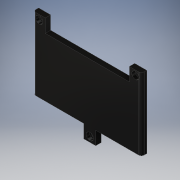
# Autodesk Inventor part: battery_cover
Saved by Autodesk Inventor 2019.4 (Build 234330000, 330)
## iProperties
Created: 2020-07-20
Part Number: battery_cover
Material: Generic
Document SubType Name: Modeling
Designer: alex_
Density: 1 g/cm^3
Appearance: Smooth - Black
Author: alex_
## iProperties of the stored document _3DPrint.ipt
Created: 2020-07-20
Part Number: _3DPrint
Material: Generic
Document SubType Name: Modeling
Designer: alex_
Density: 1 g/cm^3
Appearance: Default
Author: alex_
Autodesk Inventor part; units mm, degrees
ref_plane "YZ Plane" through (0, 0, 0) normal (1, 0, 0) x (0, 1, 0)
ref_plane "XZ Plane" through (0, 0, 0) normal (0, 1, 0) x (-1, 0, 0)
ref_plane "XY Plane" through (0, 0, 0) normal (0, 0, 1) x (1, 0, 0)
sketch "Sketch1" plane through (0, 0, 0) normal (0, 0, 1) x (1, 0, 0)
  line L0 (82, 0) -> (82, 45)
  line L1 (0, 45) -> (0, 0)
  line L2 (10, 45) -> (10, 55)
  line L3 (10, 55) -> (0, 55)
  line L4 (0, 55) -> (0, 45)
  line L5 (72, 45) -> (72, 55)
  line L6 (72, 55) -> (82, 55)
  line L7 (82, 55) -> (82, 45)
  line L8 (10, 45) -> (72, 45)
  line L9 (0, 0) -> (37.791, 0)
  line L10 (37.791, 0) -> (37.791, -10)
  line L11 (37.791, -10) -> (47.791, -10)
  line L12 (47.791, -10) -> (47.791, 0)
  line L13 (47.791, 0) -> (82, 0)
  circle A0 centre (42.843, -5.687) radius 1.6
  line L14 (0, 45) -> (0, 51)
  line L15 (82, 45) -> (82, 51)
  circle A1 centre (4.971, 51) radius 1.6
  circle A2 centre (77.029, 51) radius 1.6
  dimension "d0" = 82
  dimension "d1" = 45
  dimension "d2" = 10
  dimension "d3" = 10
  dimension "d4" = 10
  dimension "d5" = 10
  dimension "d10" = 37.791
  dimension "d11" = 10
  dimension "d12" = 10
  dimension "d15" = 3.2
  dimension "d16" = 6
  dimension "d20" = 3.2
  dimension "d21" = 3.2
  constraints: 32 end point, 4 perpendicular, 3 centre point, 3 parallel, 3 point on line, 2 horizontal
  measures "d0" distance of L1.start L0.end
  measures "d1" distance of L0.end L0.start
  measures "d2" distance of L3.end L2.end
  measures "d3" distance of L2.end L2.start
  measures "d4" distance of L5.end L6.end
  measures "d5" distance of L5.start L5.end
  measures "d10" distance of L1.end L9.end
  measures "d11" distance of L9.end L10.end
  measures "d12" distance of L10.end L11.end
  measures "d15" diameter of A0
  measures "d16" distance of L1.start L14.end
  measures "d20" diameter of A1
  measures "d21" diameter of A2
extrude "Extrusion1" add sketch "Sketch1" along normal blind 4
sketch "Sketch3" plane through (0, 0, 4) normal (0, 0, 1) x (1, 0, 0)
  circle A0 centre (4.971, 51) radius 1.6 projected
  circle A1 centre (4.971, 51) radius 2.75
  circle A2 centre (77.029, 51) radius 1.6 projected
  circle A3 centre (77.029, 51) radius 2.75
  circle A4 centre (42.843, -5.687) radius 1.6 projected
  circle A5 centre (42.843, -5.687) radius 2.75
  point P0 (0, 0)
  dimension "d24" = 5.5
  dimension "d25" = 5.5
  dimension "d26" = 5.5
  constraints: 3 centre point, 3 coincident
  measures "d24" diameter of A1
  measures "d25" diameter of A3
  measures "d26" diameter of A5
extrude "Extrusion2" cut sketch "Sketch3" against normal blind 2.5
sketch "Sketch4" plane through (0, 0, 4) normal (0, 0, 1) x (1, 0, 0)
  line L0 (10, 55) -> (0, 55) projected
  line L1 (10, 45) -> (10, 55) projected
  line L2 (0, 55) -> (10, 55)
  line L3 (10, 55) -> (10, 54.5)
  line L4 (10, 54.5) -> (0, 54.5)
  line L5 (0, 54.5) -> (0, 55)
  line L6 (0, 0) -> (0, 55) projected
  line L7 (0, 0) -> (37.791, 0) projected
  line L8 (0, 55) -> (0.5, 55)
  line L9 (0.5, 55) -> (0.5, 0)
  line L10 (0.5, 0) -> (0, 0)
  line L11 (0, 0) -> (0, 55)
  line L12 (0, 0) -> (37.791, 0)
  line L13 (37.791, 0) -> (37.791, 0.5)
  line L14 (37.791, 0.5) -> (0, 0.5)
  line L15 (0, 0.5) -> (0, 0)
  line L16 (37.791, 0) -> (37.791, -10) projected
  line L17 (37.791, -10) -> (38.291, -10)
  line L18 (38.291, -10) -> (38.291, 0.5)
  line L19 (38.291, 0.5) -> (37.791, 0.5)
  line L20 (37.791, 0.5) -> (37.791, -10)
  line L21 (47.791, 0) -> (47.791, -10) projected
  line L22 (37.791, -10) -> (47.791, -10)
  line L23 (47.791, -10) -> (47.791, -9.5)
  line L24 (47.791, -9.5) -> (37.791, -9.5)
  line L25 (37.791, -9.5) -> (37.791, -10)
  line L26 (47.791, -10) -> (47.291, -10)
  line L27 (47.291, -10) -> (47.291, 0.5)
  line L28 (47.291, 0.5) -> (47.791, 0.5)
  line L29 (47.791, 0.5) -> (47.791, -10)
  line L30 (82, 0) -> (82, 55) projected
  line L31 (47.291, 0.5) -> (82, 0.5)
  line L32 (82, 0.5) -> (82, 0)
  line L33 (82, 0) -> (47.291, 0)
  line L34 (47.291, 0) -> (47.291, 0.5)
  line L35 (82, 55) -> (72, 55) projected
  line L36 (82, 0) -> (81.5, 0)
  line L37 (81.5, 0) -> (81.5, 55)
  line L38 (81.5, 55) -> (82, 55)
  line L39 (82, 55) -> (82, 0)
  line L40 (72, 55) -> (72, 45) projected
  line L41 (82, 55) -> (72, 55)
  line L42 (72, 55) -> (72, 54.5)
  line L43 (72, 54.5) -> (82, 54.5)
  line L44 (82, 54.5) -> (82, 55)
  line L45 (10, 45) -> (72, 45) projected
  line L46 (10, 45) -> (72, 45)
  line L47 (72, 45) -> (72, 44.5)
  line L48 (72, 44.5) -> (10, 44.5)
  line L49 (10, 44.5) -> (10, 45)
  line L50 (72, 44.5) -> (72.5, 44.5)
  line L51 (72.5, 44.5) -> (72.5, 55)
  line L52 (72.5, 55) -> (72, 55)
  line L53 (72, 55) -> (72, 44.5)
  line L54 (10, 44.5) -> (9.5, 44.5)
  line L55 (9.5, 44.5) -> (9.5, 55)
  line L56 (9.5, 55) -> (10, 55)
  line L57 (10, 55) -> (10, 44.5)
  dimension "d30" = 0.5
  dimension "d31" = 0.5
  dimension "d32" = 0.5
  dimension "d33" = 0.5
  dimension "d34" = 0.5
  dimension "d35" = 0.5
  dimension "d36" = 0.5
  dimension "d37" = 0.5
  dimension "d38" = 0.5
  dimension "d39" = 0.5
  dimension "d40" = 0.5
  constraints: 96 end point, 24 parallel, 12 horizontal, 12 perpendicular, 9 point on line
  measures "d30" distance of L2.end L3.end
  measures "d31" distance of L9.end L10.end
  measures "d32" distance of L13.end L12.end
  measures "d33" distance of L19.end L18.end
  measures "d34" distance of L23.end L22.end
  measures "d35" distance of L27.end L28.end
  measures "d36" distance of L37.end L38.end
  measures "d37" distance of L42.end L41.end
  measures "d38" distance of L46.end L47.end
  measures "d39" distance of L52.end L51.end
  measures "d40" distance of L55.end L56.end
extrude "Extrusion3" cut sketch "Sketch4" against normal blind 10 contours L1 L4 L55 L0 | L55 L4 L9 L0 | L1 L49 L54 L55 L4 | L9 L4 L5 L0 | L45 L47 L48 L49 | L9 L14 L6 L4 | L40 L43 L51 L50 L47 | L14 L13 L7 L9 | L9 L7 L6 L14 | L40 L35 L51 L43 | L19 L18 L24 L16 L13 | L51 L35 L37 L43 | L43 L30 L31 L37 | L37 L35 L30 L43 | L24 L18 L17 L16 | L24 L27 L22 L18 | L37 L33 L29 L31 | L31 L30 L33 L37 | L27 L33 L21 L24 | L24 L21 L22 L27 | L29 L33 L27 L28
fillet "Fillet2" radius 2 2 edges at (0.5, 27.5, 4) (81.5, 27.5, 4)
body "Solid1"
